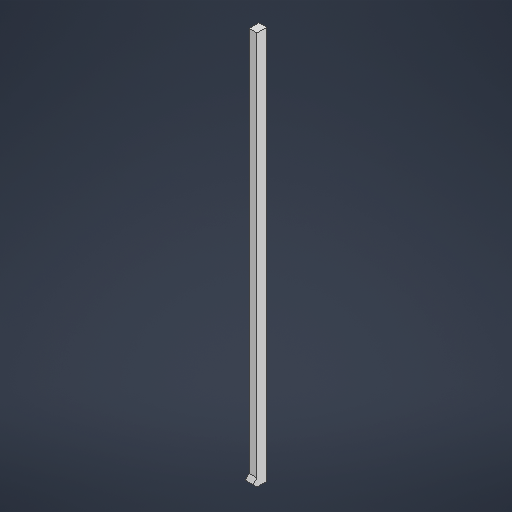
# Autodesk Inventor part: startopactutorarm
Saved by Autodesk Inventor 2026.1 (Build 301233020, 233B)
## iProperties
Created: 2025-12-12
Part Number: startopactutorarm
Material: Generic
Document SubType Name: Modeling
Designer: alexa
Density: 1 g/cm^3
Appearance: Default
Author: alexa
Autodesk Inventor part; units mm, degrees
ref_plane "YZ Plane" through (0, 0, 0) normal (1, 0, 0) x (0, 1, 0)
ref_plane "XZ Plane" through (0, 0, 0) normal (0, 1, 0) x (-1, 0, 0)
ref_plane "XY Plane" through (0, 0, 0) normal (0, 0, 1) x (1, 0, 0)
sketch "Sketch1" plane through (0, 0, 0) normal (0, 1, 0) x (-1, 0, 0)
  line L0 (0, 0) -> (4, 0)
  line L1 (4, 0) -> (4, -5)
  line L2 (4, -5) -> (0, -5)
  line L3 (0, -5) -> (0, 0)
  dimension "d0" = 4
  dimension "d1" = 5
  constraints: 8 end point, 2 parallel, 1 horizontal, 1 perpendicular
  measures "d0" distance of L1.end L2.end
  measures "d1" distance of L0.end L1.end
extrude "Extrusion1" add sketch "Sketch1" along normal blind 200
sketch "Sketch2" plane through (0, 0, 0) normal (0, 0, 1) x (1, 0, 0)
  line L0 (0, 0) -> (0, 200) projected
  line L1 (-4, 0) -> (-4, 200) projected
  line L2 (0, 0) -> (-4, 0)
  line L3 (-4, 0) -> (-4, 4)
  line L4 (-4, 4) -> (0, 4)
  line L5 (0, 4) -> (0, 0)
  dimension "d4" = 4
  constraints: 8 end point, 2 parallel, 1 horizontal, 1 perpendicular, 1 point on line
  measures "d4" distance of L2.end L3.end
extrude "Extrusion2" add sketch "Sketch2" along normal blind 2
sketch "Sketch3" plane through (0, 0, -5) normal (1, 0, 0) x (0, 0, -1)
  line L0 (-5, 4) -> (-7, 4) projected
  line L1 (-7, 4) -> (-7, 0) projected
  line L2 (-7, 4) -> (-7, 0)
  line L3 (-7, 0) -> (-7, 2)
  line L4 (-7, 2) -> (-5, 4)
  line L5 (-7, 2) -> (-5, 0)
  line L6 (0, 0) -> (-7, 0) projected
  line L7 (-5, 0) -> (-7, 0)
  line L8 (-7, 0) -> (-7, 2)
  line L9 (-7, 2) -> (-7, 4)
  line L10 (-7, 4) -> (-5, 4)
  dimension "d7" = 2
  constraints: 16 end point, 4 collinear, 2 perpendicular, 1 midpoint
  measures "d7" distance of L2.end L3.end
extrude "Extrusion3" cut sketch "Sketch3" against normal blind 4 contours L5 L6 L1
sketch "Sketch4" plane through (0, 0, -5) normal (1, 0, 0) x (0, 0, -1)
  line L0 (-5, 4) -> (-5, 200) projected
  line L1 (-7, 2) -> (-7, 4) projected
  line L2 (-5, 4) -> (-7, 2)
  line L3 (-5, 4) -> (-7, 4) projected
  line L4 (-7, 2) -> (-7, 4)
  line L5 (-7, 4) -> (-5, 4)
  line L6 (-5, 4) -> (-7, 2)
  line L7 (-7, 2) -> (-7, 4)
  point P0 (-5, 0)
  constraints: 10 end point, 2 collinear, 2 perpendicular
extrude "Extrusion4" cut sketch "Sketch4" against normal blind 4
body "Solid1"
